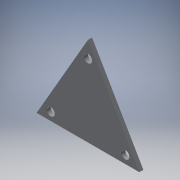
# Autodesk Inventor part: part4
Saved by Autodesk Inventor 2016 (Build 200138000, 138)
## iProperties
Created: 2017-09-07
Part Number: part4
Material: Generic
Document SubType Name: Modeling
Designer: student
Density: 1 g/cm^3
Appearance: Default
Author: student
Autodesk Inventor part; units mm, degrees
ref_plane "YZ Plane" through (0, 0, 0) normal (1, 0, 0) x (0, 1, 0)
ref_plane "XZ Plane" through (0, 0, 0) normal (0, 1, 0) x (-1, 0, 0)
ref_plane "XY Plane" through (0, 0, 0) normal (0, 0, 1) x (1, 0, 0)
sketch "Sketch1" plane through (0, 0, 0) normal (0, 0, 1) x (1, 0, 0)
  line L0 (-100.0259, 156.5662) -> (-80.9759, 123.5707) construction
  line L1 (-80.9759, 123.5707) -> (-119.0759, 123.5707) construction
  line L2 (-119.0759, 123.5707) -> (-100.0259, 156.5662) construction
  circle A0 centre (-119.0759, 123.5707) radius 3.175
  circle A1 centre (-80.9759, 123.5707) radius 3.175
  circle A2 centre (-100.0259, 156.5662) radius 3.175
  line L3 (-100.0259, 156.5662) -> (-100.0259, 169.2662) construction
  line L4 (-100.0259, 169.2662) -> (-69.9774, 117.2207)
  line L5 (-69.9774, 117.2207) -> (-130.0744, 117.2207)
  line L6 (-130.0744, 117.2207) -> (-100.0259, 169.2662)
  point P0 (0, 0)
  point P1 (-100.0259, 134.5692)
  point P2 (-100.0259, 134.5692)
  dimension "d12" = 38.1
  dimension "d13" = 6.35
  dimension "d14" = 6.35
  dimension "d15" = 6.35
  dimension "d17" = 12.7
  constraints: 14 end point, 4 coincident, 3 centre point, 1 vertical, 14 other
  measures "d12" distance of L0.end L1.end
  measures "d13" diameter of A0
  measures "d14" diameter of A1
  measures "d15" diameter of A2
  measures "d17" distance of L3.start L3.end
extrude "Extrusion1" add sketch "Sketch1" along normal blind 3.175
body "Solid1"
